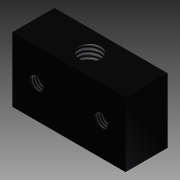
# Autodesk Inventor part: PS20010
Saved by Autodesk Inventor 2014 (Build 180170000, 170)
## iProperties
Company: Shapeoko LLC
Category: NS
Created: 2012-04-26
Part Number: PS20010
Material: Acetal Resin, Black
Document SubType Name: Modeling
Designer: ERF
Mass: 11.4812 g
Surface Area: 34.6222 cm^2
Volume: 8.057 cm^3
Density: 1.425 g/cm^3
Project: Shapeoko
Vendor: Netbeef
Engineer: ERF
Checked By: Edward
Engr Approved By: Edward
Description: 13mm x 35mm x 20mm Delrin Lead nut
Stock Number: SM-M08
Appearance: Smooth - Black
User Status: F
Authority: NEED QUOTE FROM NETBEEF FOR PRICE
Title: Delrin lead nut.
Subject: Motion
Author: ERF
Revision Number: 3
Comments: Inventables
Autodesk Inventor part; units mm, degrees
ref_plane "YZ Plane" through (0, 0, 0) normal (1, 0, 0) x (0, 1, 0)
ref_plane "XZ Plane" through (0, 0, 0) normal (0, 1, 0) x (-1, 0, 0)
ref_plane "XY Plane" through (0, 0, 0) normal (0, 0, 1) x (1, 0, 0)
sketch "Sketch1" plane through (0, 0, 0) normal (0, 0, 1) x (1, 0, 0)
  line L0 (-17.5, 10) -> (17.5, 10)
  line L1 (17.5, 10) -> (17.5, -10)
  line L2 (17.5, -10) -> (-17.5, -10)
  line L3 (-17.5, -10) -> (-17.5, 10)
  point P0 (0, 0)
  dimension "d0" = 35
  dimension "d1" = 20
  dimension "d2" = 10
  dimension "d3" = 17.5
  constraints: 8 end point, 2 parallel, 1 horizontal, 1 perpendicular
  measures "d0" distance of L1.end L2.end
  measures "d1" distance of L0.end L1.end
  measures "d2" distance from line of L0 point (0, 0)
  measures "d3" distance from line of point (0, 0) L3
extrude "Extrusion1" add sketch "Sketch1" along normal blind 13
sketch "Sketch2" plane through (0, 0, 13) normal (0, 0, 1) x (1, 0, 0)
  line L0 (-17.5, 10) -> (17.5, 10) projected
  line L1 (-17.5, -10) -> (-17.5, 10) projected
  circle A0 centre (-10, 0) radius 2.1
  circle A1 centre (10, 0) radius 2.1
  point P0 (0, 0)
  dimension "d6" = 4.2
  dimension "d7" = 4.2
  dimension "d8" = 20
  dimension "d9" = 10
  dimension "d10" = 10
  dimension "d11" = 7.5
  constraints: 2 centre point
  measures "d6" diameter of A0
  measures "d7" diameter of A1
  measures "d8" distance of A1.centre A0.centre
  measures "d9" distance from line of L0 A0.centre
  measures "d10" distance from line of L0 A1.centre
  measures "d11" distance from line of L1 A0.centre
hole "Hole1" at (-10, 0, 13) at (10, 0, 13) direction (0, 0, -1) diameter 4.134 end through all thread size "M5x0.8" class "6H" standard "ANSI Metric M Profile"
sketch "Sketch3" plane through (-17.5, 10, 0) normal (0, 1, 0) x (1, 0, 0)
  line L0 (0, 0) -> (35, 0) projected
  line L1 (0, 0) -> (0, -13) projected
  circle A0 centre (17.5, -6.5) radius 3.375
  point P0 (17.5, 0)
  dimension "d19" = 6.75
  dimension "d20" = 17.5
  dimension "d21" = 6.5
  constraints: 1 centre point
  measures "d19" diameter of A0
  measures "d20" distance from line of L1 A0.centre
  measures "d21" distance from line of L0 A0.centre
hole "Hole2" at (0, 10, 6.5) direction (0, -1, 0) diameter 6.647 end through all thread size "M8x1.25" class "6H" standard "ANSI Metric M Profile"
equation "\"d2\" = 0.5 * d1"
equation "\"d3\" = 0.5 * d0"
body "Solid1"
